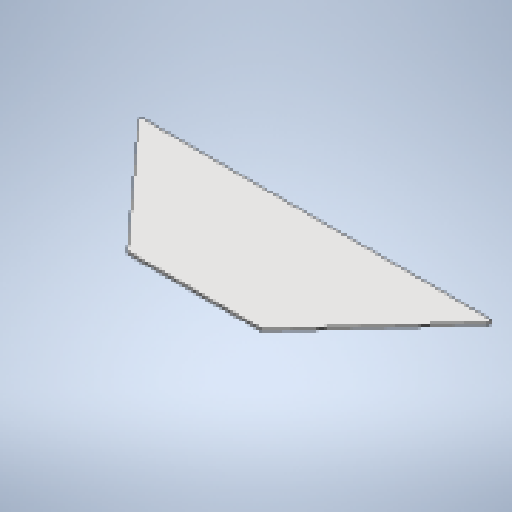
# Autodesk Inventor part: ДМФ 052 торец лотка кормовой v2.0
Saved by Autodesk Inventor 2026.2 (Build 302298010, 298A)
## iProperties
Created: 2024-05-13
Part Number: ДМФ 052 торец лотка кормовой v2.0
Material: Generic
Document SubType Name: Sheet Metal
Designer: admin
Density: 1 g/cm^3
Sheet Metal Rule: Default
Appearance: Default
Mass: 72.5735 g
Surface Area: 505.677 cm^2
Volume: 72.5735 cm^3
Flat Pattern Width: 11 cm
Flat Pattern Length: 31.4958 cm
Flat Pattern Area: 346.454 cm^2
Sheet Metal Width: 110,000 mm
Sheet Metal Length: 314,958 mm
Sheet Metal Area: 34645,357 mm^2
Author: admin
Autodesk Inventor part; units mm, degrees
ref_plane "YZ Plane" through (0, 0, 0) normal (1, 0, 0) x (0, 1, 0)
ref_plane "XZ Plane" through (0, 0, 0) normal (0, 1, 0) x (-1, 0, 0)
ref_plane "XY Plane" through (0, 0, 0) normal (0, 0, 1) x (1, 0, 0)
sketch "Sketch1" plane through (0, 0, 0) normal (0, 0, 1) x (1, 0, 0)
  line L0 (-160, 110) -> (-60, 0)
  line L1 (-60, 0) -> (60, 0)
  line L2 (60, 0) -> (160, 110)
  line L3 (160, 110) -> (-160, 110)
  point P0 (0, 0)
  point P1 (0, 0)
  point P2 (0, 110)
  dimension "d0" = 110
  dimension "d1" = 120
  dimension "d2" = 320
  measures "d0" distance between parallel lines of L1 L3
  measures "d1" distance of L0.end L1.end
  measures "d2" distance of L2.end L0.start
extrude "Plate1" add sketch "Sketch1" along normal blind 2
fillet "Corner Round1" radius 2 2 edges at (160, 110, 1) (-160, 110, 1)
equation "\"d3\" = Thickness"
equation "\"BendRadius\" = Thickness"
equation "\"BendReliefWidth\" = Thickness"
equation "\"BendReliefDepth\" = 0.5 * Thickness"
equation "\"CornerReliefSize\" = 4 * Thickness"
equation "\"MinimumRemnant\" = 2 * Thickness"
equation "\"TransitionRadius\" = BendRadius"
equation "\"JacobiRadiusSize\" = BendRadius"
equation "\"GapSize\" = Thickness"
equation "\"Thickness\" = 2"
body "Solid1"
